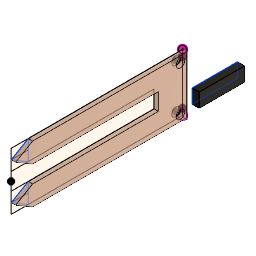
Irrigation unit - soil humidity sensor v1 (Autodesk Fusion 360 design; units mm, degrees)
Autodesk Fusion 360 part; units mm, degrees
sketch "Sketch1" plane through (0, 0, 0) normal (1, 0, 0) x (0, 0, -1)
  line L0 (0, 0) -> (20, 0)
  line L1 (20, 0) -> (20, -60)
  line L2 (20, -60) -> (0, -60)
  line L3 (0, -60) -> (0, 0)
  line L4 (7, -10) -> (13, -10)
  line L5 (13, -10) -> (13, -60)
  line L6 (13, -60) -> (7, -60)
  line L7 (7, -60) -> (7, -10)
  line L8 (0, -54) -> (7, -54)
  line L9 (13, -54) -> (20, -54)
  line L10 (3.5, -54) -> (3.5, -60)
  line L11 (16.5, -54) -> (16.5, -60)
  line L12 (16.5, -60) -> (13, -54)
  line L13 (16.5, -60) -> (20, -54)
  line L14 (3.5, -60) -> (0, -54)
  line L15 (3.5, -60) -> (7, -54)
  circle A0 centre (2.2, -2.25) radius 1.5
  circle A1 centre (17.8, -2.25) radius 1.5
  dimension "d46" = 60
  dimension "d47" = 20
  dimension "d48" = 6
  dimension "d49" = 50
  dimension "d51" = 3
  dimension "d52" = 2.25
  dimension "d53" = 2.2
  dimension "d54" = 3
  dimension "d55" = 2.25
  dimension "d56" = 2.2
  measures "d51" diameter of A0
  measures "d54" diameter of A1
extrude "Extrude1" add sketch "Sketch1" along normal blind 1.55 contours L0 L1 L3 L4 L5 L7 L8 L9 | L8 L10 L14 | L9 L11 L13 | L8 L10 L15 | L9 L11 L12 makes body 1
ref_plane "WorkPlane1" through (6.05, -30, -10) normal (1, 0, 0) x (0, 0, -1)
sketch "Sketch2" plane through (6.05, -30, -10) normal (1, 0, 0) x (0, 0, -1)
  line L0 (-2.7003, 27.3001) -> (2.2997, 27.3001)
  line L1 (2.2997, 27.3001) -> (2.2997, 43.3001)
  line L2 (2.2997, 43.3001) -> (-2.7003, 43.3001)
  line L3 (-2.7003, 43.3001) -> (-2.7003, 27.3001)
  dimension "d60" = 5
  dimension "d61" = 16
extrude "Extrude2" add sketch "Sketch2" along normal blind 2.5 separate body makes body 2
sketch "used for creating hole in the outer box" plane through (0, 0, 0) normal (0, 1, 0) x (-1, 0, 0)
  line L0 (0, -20) -> (0, 0)
  line L1 (0, 0) -> (-1.55, 0)
  line L2 (-1.55, 0) -> (-1.55, -20)
  line L3 (-1.55, -20) -> (0, -20)
  line L4 (-1.55, -20.5) -> (0, -20.5)
  line L5 (0, -20.5) -> (0, 0.5)
  line L6 (0, 0.5) -> (-1.55, 0.5)
  line L7 (-1.55, 0.5) -> (-1.55, -20.5)
  line L8 (0, 0) -> (0, -20)
  dimension "d181" = 0.5
  dimension "d182" = 0.5
  measures "d181" distance of L3 L4
  measures "d182" distance of L1 L6
